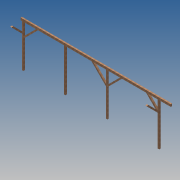
# Autodesk Inventor part: highSide
Saved by Autodesk Inventor 2013 (Build 170138000, 138)
## iProperties
Created: 2013-08-10
Part Number: highSide
Material: Wood (Birch)
Document SubType Name: Modeling
Designer: ddeboer
Mass: 130094 g
Surface Area: 96157.3 cm^2
Volume: 236534 cm^3
Density: 0.55 g/cm^3
Author: ddeboer
Autodesk Inventor part; units mm, degrees
ref_plane "YZ Plane" through (0, 0, 0) normal (1, 0, 0) x (0, 1, 0)
ref_plane "XZ Plane" through (0, 0, 0) normal (0, 1, 0) x (-1, 0, 0)
ref_plane "XY Plane" through (0, 0, 0) normal (0, 0, 1) x (1, 0, 0)
sketch "Sketch1" plane through (0, 0, 0) normal (0, 0, 1) x (1, 0, 0)
  line L0 (0, 0) -> (88.9, 0)
  line L1 (88.9, 0) -> (88.9, 2654.3)
  line L2 (88.9, 2654.3) -> (0, 2654.3)
  line L3 (0, 2654.3) -> (0, 0)
  line L4 (44.45, 2654.3) -> (806.45, 2654.3) construction
  line L5 (806.45, 2654.3) -> (-8566.15, 2654.3)
  line L6 (-8566.15, 2654.3) -> (-8566.15, 2794)
  line L7 (-8566.15, 2794) -> (806.45, 2794)
  line L8 (806.45, 2794) -> (806.45, 2654.3)
  line L9 (-3143.25, 0) -> (-3232.15, 0)
  line L10 (-3232.15, 0) -> (-3232.15, 2654.3)
  line L11 (-3232.15, 2654.3) -> (-3143.25, 2654.3)
  line L12 (-3143.25, 2654.3) -> (-3143.25, 0)
  line L13 (-5759.45, 0) -> (-5848.35, 0)
  line L14 (-5848.35, 0) -> (-5848.35, 2654.3)
  line L15 (-5848.35, 2654.3) -> (-5759.45, 2654.3)
  line L16 (-5759.45, 2654.3) -> (-5759.45, 0)
  line L17 (-8382, 0) -> (-8470.9, 0)
  line L18 (-8470.9, 0) -> (-8470.9, 2654.3)
  line L19 (-8470.9, 2654.3) -> (-8382, 2654.3)
  line L20 (-8382, 2654.3) -> (-8382, 0)
  line L21 (0, 1892.3) -> (-764.7126, 2657.0126)
  line L22 (0, 1892.3) -> (1081.4669, 1892.3) construction
  line L23 (-62.8618, 1829.4382) -> (-827.5744, 2594.1508)
  line L24 (-827.5744, 2594.1508) -> (-887.7236, 2654.3)
  line L25 (-62.8618, 1829.4382) -> (0, 1766.5764)
  line L26 (-3232.15, 1870.9072) -> (-3996.8615, 2635.6187)
  line L27 (-3295.0107, 1808.0443) -> (-4059.7233, 2572.7569)
  line L28 (-3295.0107, 1808.0443) -> (-3232.15, 1745.1837)
  line L29 (-4059.7233, 2572.7569) -> (-4141.2663, 2654.3)
  line L30 (-3996.8615, 2635.6187) -> (-4015.5428, 2654.3)
  line L31 (-3187.7, 2654.3) -> (-3187.7, 0) construction
  line L32 (-3232.15, 1745.1837) -> (-3232.15, 1870.9072)
  line L33 (-4141.2663, 2654.3) -> (-4015.5428, 2654.3)
  line L34 (-3143.25, 1870.9072) -> (-2378.5385, 2635.6187)
  line L35 (-3080.3893, 1808.0443) -> (-2315.6767, 2572.7569)
  line L36 (-3080.3893, 1808.0443) -> (-3143.25, 1745.1837)
  line L37 (-2315.6767, 2572.7569) -> (-2234.1337, 2654.3)
  line L38 (-2378.5385, 2635.6187) -> (-2359.8572, 2654.3)
  line L39 (-3143.25, 1745.1837) -> (-3143.25, 1870.9072)
  line L40 (-2234.1337, 2654.3) -> (-2359.8572, 2654.3)
  line L41 (-7554.4267, 2572.7569) -> (-7472.8837, 2654.3)
  line L42 (-7617.2885, 2635.6187) -> (-7598.6072, 2654.3)
  line L43 (-8382, 1870.9072) -> (-7617.2885, 2635.6187)
  line L44 (-8319.1393, 1808.0443) -> (-7554.4267, 2572.7569)
  line L45 (-8319.1393, 1808.0443) -> (-8382, 1745.1837)
  line L46 (-8382, 1745.1837) -> (-8382, 1870.9072)
  dimension "d0" = 88.9
  dimension "d1" = 2654.3
  dimension "d2" = 762
  dimension "d3" = 9372.6
  dimension "d4" = 139.7
  dimension "d5" = 88.9
  dimension "d6" = 3232.15
  dimension "d7" = 88.9
  dimension "d8" = 2616.2
  dimension "d9" = 88.9
  dimension "d10" = 2622.55
  dimension "d11" = 135
  dimension "d12" = 762
  dimension "d13" = 88.9
  dimension "d14" = 88.9
  constraints: 92 end point, 12 parallel, 7 horizontal, 7 symmetric about line, 5 collinear, 5 perpendicular, 5 point on line, 3 midpoint, 1 equal length, 1 vertical, 11 other
  measures "d0" distance of L0.start L0.end
  measures "d1" distance of L2.end L0.start
  measures "d2" distance of L4.start L4.end
  measures "d3" distance of L4.end L6.start
  measures "d4" distance of L7.end L4.end
  measures "d5" distance of L9.start L9.end
  measures "d6" distance between parallel lines of L12 L1
  measures "d7" distance of L13.start L13.end
  measures "d8" distance between parallel lines of L16 L12
  measures "d9" distance of L17.start L17.end
  measures "d10" distance between parallel lines of L20 L16
  measures "d11" angle of L22 L21
  measures "d12" distance of L2.end L21.start
  measures "d13" distance between parallel lines of L23 L21
  measures "d14" distance between parallel lines of L27 L26
extrude "Extrusion1" add sketch "Sketch1" along normal blind 88.9 contours L3 L2 L1 L0 | L2 L5 L6 L7 L8 | L37 L35 L36 L12 L34 L38 L5 | L5 L20 L17 L18 | L12 L9 L10 L5 | L5 L41 L44 L45 L20 L43 L42 | L30 L26 L10 L28 L27 L29 L5 | L5 L16 L13 L14
sketch "Sketch2" plane through (0, 0, 88.9) normal (0, 0, 1) x (1, 0, 0)
  line L0 (-2234.1337, 2654.3) -> (0, 2654.3) projected
  line L1 (0, 2654.3) -> (0, 0) projected
  line L2 (0, 2053.9959) -> (-600.3041, 2654.3)
  line L3 (0, 2053.9959) -> (848.9582, 2053.9959) construction
  line L4 (-666.5241, 2588.0801) -> (-38.7907, 1960.3467)
  line L5 (-38.7907, 1960.3467) -> (0, 1921.556)
  line L6 (-666.5241, 2588.0801) -> (-732.744, 2654.3)
  dimension "d17" = 135
  constraints: 10 end point, 4 point on line, 2 collinear, 1 equal length, 1 horizontal
  measures "d17" angle of L3 L2
extrude "Extrusion2" add sketch "Sketch2" against normal blind 88.9 contours L0 L2 L1 L5 L4 L6
sketch "Sketch3" plane through (0, 0, 0) normal (0, -1, 0) x (1, 0, 0)
  circle A0 centre (44.45, 44.45) radius 12.7
  dimension "d20" = 25.4
  constraints: 1 centre point
  measures "d20" diameter of A0
extrude "Extrusion3" cut sketch "Sketch3" against normal blind 25.4
sketch "Sketch4" plane through (88.9, 0, 0) normal (1, 0, 0) x (0, 0, -1)
  line L0 (-88.9, 0) -> (-88.9, 2654.3) projected
  line L1 (-88.9, 2059.8437) -> (-763.3688, 2734.3125)
  line L2 (-88.9, 2059.8437) -> (1181.1, 2059.8437) construction
  line L3 (-877.1351, 2722.3552) -> (-111.7219, 1956.942)
  line L4 (-111.7219, 1956.942) -> (-88.9, 1934.1201)
  line L5 (-1112.6492, 2957.8693) -> (-986.9256, 2957.8693)
  line L6 (-88.9, 2059.8437) -> (-88.9, 1934.1201)
  line L7 (-763.3688, 2734.3125) -> (-877.1351, 2722.3552)
  line L8 (-840.5667, 2926.4384) -> (-285.5134, 2926.4384) construction
  line L9 (-88.9, 2147.6306) -> (-717.5179, 2776.2485) construction
  line L10 (-88.9, 2147.6306) -> (800.1, 2147.6306) construction
  point P0 (-1081.2183, 2926.4384)
  dimension "d23" = 1270
  dimension "d24" = 135
  dimension "d25" = 88.9
  dimension "d34" = 174
  dimension "d35" = 889
  dimension "d36" = 135
  constraints: 20 end point, 4 point on line, 3 horizontal, 2 collinear, 1 equal length, 1 parallel
  measures "d23" distance of L1.start L5.end
  measures "d24" angle of L2 L1
  measures "d25" distance between parallel lines of L3 L1
  measures "d34" angle of L7 L8
  measures "d35" distance of L9.start L9.end
  measures "d36" angle of L10 L9
extrude "Extrusion4" add sketch "Sketch4" against normal blind 88.9
sketch "Sketch5" plane through (-8470.9, 0, 0) normal (-1, 0, 0) x (0, 0, 1)
  line L0 (88.9, 2654.3) -> (88.9, 0) projected
  line L1 (88.9, 2100.9628) -> (717.5179, 2729.5808)
  line L2 (88.9, 2100.9628) -> (977.9, 2100.9628) construction
  line L3 (831.2842, 2717.6234) -> (293.7757, 2180.1149)
  line L4 (293.7757, 2180.1149) -> (88.9, 1975.2392)
  line L5 (717.5179, 2729.5808) -> (843.2415, 2729.5808)
  line L6 (88.9, 1975.2392) -> (88.9, 2100.9628)
  line L7 (717.5179, 2729.5808) -> (831.2842, 2717.6234)
  line L8 (843.2415, 2729.5808) -> (937.1256, 2729.5808) construction
  dimension "d28" = 889
  dimension "d29" = 45
  dimension "d30" = 88.9
  dimension "d33" = 6
  constraints: 16 end point, 2 collinear, 2 horizontal, 2 point on line, 1 equal length, 1 parallel
  measures "d28" distance of L1.start L1.end
  measures "d29" angle of L2 L1
  measures "d30" distance between parallel lines of L3 L1
  measures "d33" angle of L7 L8
extrude "Extrusion5" add sketch "Sketch5" against normal blind 88.9
body "Solid1"
